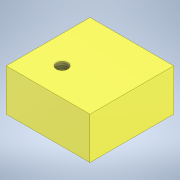
# Autodesk Inventor part: Soporte_Base_Madera
Saved by Autodesk Inventor 2022 (Build 260153000, 153)
## iProperties
Created: 2022-01-24
Part Number: Soporte_Base_Madera
Material: PC/ABS Plastic
Document SubType Name: Modeling
Designer: hurta
Density: 0.357273 g/cm^3
Appearance: Smooth - Yellow
Author: hurta
Autodesk Inventor part; units mm, degrees
ref_plane "YZ Plane" through (0, 0, 0) normal (1, 0, 0) x (0, 1, 0)
ref_plane "XZ Plane" through (0, 0, 0) normal (0, 1, 0) x (-1, 0, 0)
ref_plane "XY Plane" through (0, 0, 0) normal (0, 0, 1) x (1, 0, 0)
sketch "Sketch1" plane through (0, 0, 0) normal (0, 1, 0) x (-1, 0, 0)
  line L0 (15, -15) -> (-15, -15)
  line L1 (-15, -15) -> (-15, 15)
  line L2 (-15, 15) -> (15, 15)
  line L3 (15, 15) -> (15, -15)
  line L4 (15, -15) -> (-15, 15) construction
  line L5 (-15, -15) -> (15, 15) construction
  point P0 (0, 0)
  point P1 (5, 5)
  dimension "d0" = 30
  dimension "d1" = 30
  dimension "d2" = 10
  dimension "d3" = 10
  constraints: 12 end point, 2 midpoint, 2 parallel, 1 horizontal, 1 perpendicular
  measures "d0" distance of L1.end L2.end
  measures "d1" distance of L0.end L1.end
  measures "d2" distance from line of L3 point (5, 5)
  measures "d3" distance from line of point (5, 5) L2
extrude "Extrusion1" add sketch "Sketch1" along normal blind 15
hole "Hole1" at (-5, 0, 5) direction (0, 1, 0) diameter 4.134 end through all counterbore diameter 12.24 counterbore depth 3.58 thread size "M5x0.8" class "6H" standard "ANSI Metric M Profile"
body "Solid1"
